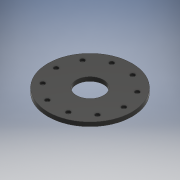
# Autodesk Inventor part: SG01
Saved by Autodesk Inventor 2017 (Build 210142000, 142)
## iProperties
Created: 2019-09-21
Part Number: SG01
Material: ABS Plastic
Document SubType Name: Modeling
Designer: Dell
Density: 1.06 g/cm^3
Appearance: Smooth - Black
Mass: 48.3343 g
Surface Area: 191.823 cm^2
Volume: 45.5984 cm^3
Author: Dell
Autodesk Inventor part; units mm, degrees
ref_plane "YZ Plane" through (0, 0, 0) normal (1, 0, 0) x (0, 1, 0)
ref_plane "XZ Plane" through (0, 0, 0) normal (0, 1, 0) x (-1, 0, 0)
ref_plane "XY Plane" through (0, 0, 0) normal (0, 0, 1) x (1, 0, 0)
sketch "Sketch1" plane through (0, 0, 0) normal (0, 0, 1) x (1, 0, 0)
  circle A0 centre (0, 0) radius 37.25
  circle A1 centre (0, 0) radius 12
  dimension "d0" = 74.5
  dimension "d1" = 24
  constraints: 2 centre point, 2 coincident
  measures "d0" diameter of A0
  measures "d1" diameter of A1
extrude "Extrusion1" add sketch "Sketch1" along normal blind 10
sketch "Sketch7" plane through (0, 0, 10) normal (0, 0, 1) x (1, 0, 0)
  circle A0 centre (0, 0) radius 22
  circle A1 centre (0, 0) radius 38
  dimension "d32" = 44
  dimension "d33" = 76
  constraints: 2 centre point, 2 coincident
  measures "d32" diameter of A0
  measures "d33" diameter of A1
extrude "Extrusion6" cut sketch "Sketch7" against normal blind 6.35 contours A0 | A1
sketch "Sketch9" plane through (0, 0, 3.65) normal (0, 0, 1) x (1, 0, 0)
  circle A0 centre (30, 0) radius 1
  circle A1 centre (24.2705, 17.6336) radius 1
  circle A2 centre (9.2705, 28.5317) radius 1
  circle A3 centre (-9.2705, 28.5317) radius 1
  circle A4 centre (-24.2705, 17.6336) radius 1
  circle A5 centre (-30, 0) radius 1
  circle A6 centre (-24.2705, -17.6336) radius 1
  circle A7 centre (-9.2705, -28.5317) radius 1
  circle A8 centre (9.2705, -28.5317) radius 1
  circle A9 centre (24.2705, -17.6336) radius 1
  point P0 (0, 0)
  dimension "d44" = 2
  dimension "d45" = 30
  dimension "d48" = 360
  constraints: 10 centre point, 1 horizontal alignment, 21 other
  measures "d44" diameter of A0
  measures "d45" distance of A0.centre point (0, 0)
extrude "Extrusion8" cut sketch "Sketch9" against normal through all
sketch "Sketch10" plane through (0, 0, 3.65) normal (0, 0, 1) x (1, 0, 0)
  circle A0 centre (30, 0) radius 1 projected
  circle A1 centre (30, 0) radius 1 projected
  circle A2 centre (30, 0) radius 2
  circle A3 centre (24.2705, 17.6336) radius 2
  circle A4 centre (9.2705, 28.5317) radius 2
  circle A5 centre (-9.2705, 28.5317) radius 2
  circle A6 centre (-24.2705, 17.6336) radius 2
  circle A7 centre (-30, 0) radius 2
  circle A8 centre (-24.2705, -17.6336) radius 2
  circle A9 centre (-9.2705, -28.5317) radius 2
  circle A10 centre (9.2705, -28.5317) radius 2
  circle A11 centre (24.2705, -17.6336) radius 2
  point P0 (0, 0)
  dimension "d52" = 4
  dimension "d55" = 360
  constraints: 10 centre point, 1 coincident, 21 other
  measures "d52" diameter of A2
extrude "Extrusion9" cut sketch "Sketch10" against normal blind 2 contours A0 | A2 | A3 | A4 | A5 | A6 | A7 | A8 | A9 | A10 | A11
body "Solid1"
